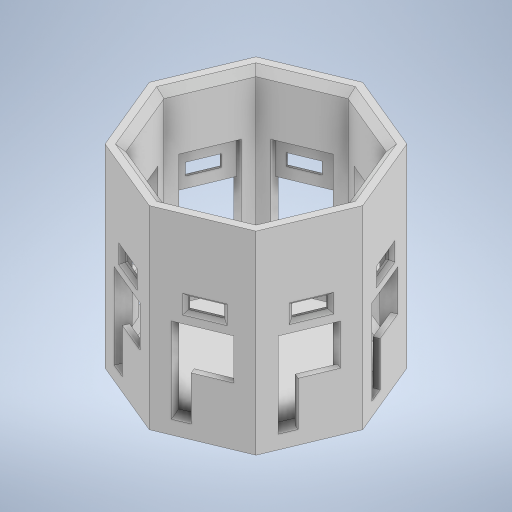
# Autodesk Inventor part: body_main
Saved by Autodesk Inventor 2023 (Build 270158000, 158)
## iProperties
Created: 2022-05-03
Part Number: body_main
Material: Ogólny
Document SubType Name: Modeling
Designer: Ciućmok
Density: 1 g/cm^3
Appearance: Domyślna
Author: Ciućmok
Autodesk Inventor part; units mm, degrees
ref_plane "YZ Plane" through (0, 0, 0) normal (1, 0, 0) x (0, 1, 0)
ref_plane "XZ Plane" through (0, 0, 0) normal (0, 1, 0) x (-1, 0, 0)
ref_plane "XY Plane" through (0, 0, 0) normal (0, 0, 1) x (1, 0, 0)
sketch "Szkic1" plane through (0, 0, 0) normal (0, 1, 0) x (-1, 0, 0)
  line L0 (0, 0) -> (0, 31.3575)
  line L1 (0, 31.3575) -> (22.1731, 22.1731)
  line L2 (22.1731, 22.1731) -> (0, 0)
  dimension "d0" = 45
  dimension "d1" = 24
  constraints: 6 end point, 1 equal length, 1 vertical
  measures "d0" angle of L2 L0
  measures "d1" distance of L0.end L1.end
extrude "Wyciągnięcie proste1" add sketch "Szkic1" along normal blind 2
sketch "Szkic2" plane through (0, 2, 0) normal (0, 1, 0) x (1, 0, 0)
  line L0 (-22.1731, -22.1731) -> (0, -31.3575) projected
  line L1 (0, 0) -> (-22.1731, -22.1731) projected
  line L2 (-19.1116, -19.1116) -> (0, -27.0279)
  line L3 (0, -31.3575) -> (0, 0) projected
  line L4 (0, -27.0279) -> (0, -31.3575)
  line L5 (-22.1731, -22.1731) -> (0, -31.3575)
  line L6 (-22.1731, -22.1731) -> (-19.1116, -19.1116)
  dimension "d4" = 4
  constraints: 8 end point, 2 point on line, 1 collinear, 1 parallel
  measures "d4" distance between parallel lines of L0 L2
extrude "Wyciągnięcie proste2" add sketch "Szkic2" along normal blind 40 contours L1 L2 L3 L0
sketch "Szkic3" plane through (-19.1116, 2, 19.1116) normal (0.3826834, 0, -0.9238795) x (-0.9238795, 0, -0.3826834)
  line L0 (-3.3304, 38) -> (-17.3304, 38)
  line L1 (-17.3304, 38) -> (-17.3304, 2)
  line L2 (-17.3304, 2) -> (-3.3304, 2)
  line L3 (-3.3304, 2) -> (-3.3304, 38)
  line L4 (1.6569, 40) -> (-22.3431, 40) construction
  line L5 (-20.6863, 0) -> (-10.3431, 0) construction
  line L6 (0.0255, 40) -> (-20.6863, 0) construction
  line L7 (-10.3431, 0) -> (0, 0) construction
  line L8 (0, 0) -> (-20.6863, 40) construction
  line L9 (-17.3304, 2) -> (-3.3304, 38) construction
  line L10 (-3.3304, 2) -> (-17.3304, 38) construction
  point P0 (-10.3431, -2)
  point P1 (-10.3304, 20)
  dimension "d7" = 14
  dimension "d8" = 36
  constraints: 16 end point, 2 midpoint, 2 parallel, 2 point on line, 1 horizontal, 1 perpendicular
  measures "d7" distance of L1.end L2.end
  measures "d8" distance of L0.end L1.end
sketch "Szkic4" plane through (0, 42, 0) normal (0, 1, 0) x (1, 0, 0)
  point P0 (0, 0)
sketch "Szkic5" plane through (0, 42, 0) normal (0, 1, 0) x (1, 0, 0)
  line L0 (0, -27.0279) -> (-19.1116, -19.1116) construction
  line L1 (-19.1116, -19.1116) -> (-22.1731, -22.1731) construction
  line L2 (-22.1731, -22.1731) -> (0, -31.3575) construction
  line L3 (0, -31.3575) -> (0, -27.0279) construction
  line L4 (-8.0251, -23.7038) -> (-9.5558, -27.3994) construction
  line L5 (-22.1731, -22.1731) -> (0, -31.3575) construction
  point P0 (0, 0)
  constraints: 2 end point, 2 point on line, 1 perpendicular
extrude "Wyciągnięcie proste3" cut sketch "Szkic3" against normal blind 2.4
sketch "Szkic6" plane through (-20.0301, 2, 21.329) normal (0.3826834, 0, -0.9238795) x (-0.9238795, 0, -0.3826834)
  line L0 (-17.3304, 2) -> (-17.3304, 38) projected
  line L1 (-3.3304, 2) -> (-17.3304, 2) projected
  line L2 (-3.3304, 38) -> (-3.3304, 2) projected
  line L3 (-17.3304, 38) -> (-3.3304, 38) projected
  line L4 (-3.3304, 38) -> (-3.3304, 2) projected
  line L5 (-17.3304, 38) -> (-3.3304, 38) projected
  line L6 (-7.7929, 2) -> (-7.7929, 27)
  line L7 (-7.7929, 27) -> (-3.3304, 27)
  line L8 (-7.7929, 27) -> (-17.3304, 27)
  line L9 (-17.3304, 2) -> (-17.3304, 38) projected
  line L10 (-17.3304, 15) -> (-7.7929, 15)
  point P0 (-10.3431, -2)
  point P1 (-17.3304, 25)
  point P2 (-17.3304, 13)
  point P3 (-3.3304, 27)
  dimension "d17" = 25
  dimension "d18" = 13
  constraints: 8 end point, 8 point on line, 2 perpendicular, 1 vertical
  measures "d17" distance of L6.start L6.end
  measures "d18" distance between parallel lines of L1 L10
extrude "Wyciągnięcie proste4" cut sketch "Szkic6" against normal through all contours L0 L8 L6 L10 | L6 L7 L2 L1
sketch "Szkic7" plane through (-20.0301, 2, 21.329) normal (0.3826834, 0, -0.9238795) x (-0.9238795, 0, -0.3826834)
  line L0 (-14.8304, 30.2) -> (-6.8304, 30.2)
  line L1 (-6.8304, 30.2) -> (-6.8304, 33.7)
  line L2 (-6.8304, 33.7) -> (-14.8304, 33.7)
  line L3 (-14.8304, 33.7) -> (-14.8304, 30.2)
  line L4 (-17.3304, 38) -> (-3.3304, 38) projected
  line L5 (-17.3304, 2) -> (-17.3304, 38) projected
  point P0 (-10.3431, -2)
  point P1 (-10.3304, 38)
  dimension "d19" = 8
  dimension "d20" = 3.5
  dimension "d21" = 4.3
  dimension "d22" = 2.5
  constraints: 8 end point, 2 parallel, 1 horizontal, 1 midpoint, 1 perpendicular
  measures "d19" distance of L2.end L1.end
  measures "d20" distance of L0.end L1.end
  measures "d21" distance from line of point (-10.33, 38) L2
  measures "d22" distance between parallel lines of L5 L3
extrude "Wyciągnięcie proste5" cut sketch "Szkic7" against normal blind 10
chamfer "Faza1" distance 1 angle 45 4 edges at (-10.6364, 35.7, 26.9518) (-14.3319, 33.95, 25.421) (-10.6364, 32.2, 26.9518) (-6.9409, 33.95, 28.4825)
pattern_circular "Szyk kołowy1" count 8 over 360 about axis through (0, 0, 0) along (0, 1, 0)
sketch "Szkic8" plane through (0, 42, 0) normal (0, 1, 0) x (1, 0, 0)
  line L0 (-22.1731, -22.1731) -> (0, -31.3575) projected
  line L1 (0, -31.3575) -> (22.1731, -22.1731) projected
  line L2 (22.1731, -22.1731) -> (31.3575, 0) projected
  line L3 (31.3575, 0) -> (22.1731, 22.1731) projected
  line L4 (22.1731, 22.1731) -> (0, 31.3575) projected
  line L5 (0, 31.3575) -> (-22.1731, 22.1731) projected
  line L6 (-22.1731, 22.1731) -> (-31.3575, 0) projected
  line L7 (-31.3575, 0) -> (-22.1731, -22.1731) projected
  line L8 (-19.1116, -19.1116) -> (-27.0279, 0) projected
  line L9 (-27.0279, 0) -> (-19.1116, 19.1116) projected
  line L10 (-19.1116, 19.1116) -> (0, 27.0279) projected
  line L11 (0, 27.0279) -> (19.1116, 19.1116) projected
  line L12 (19.1116, 19.1116) -> (27.0279, 0) projected
  line L13 (27.0279, 0) -> (19.1116, -19.1116) projected
  line L14 (19.1116, -19.1116) -> (0, -27.0279) projected
  line L15 (0, -27.0279) -> (-19.1116, -19.1116) projected
  point P0 (0, 0)
extrude "Wyciągnięcie proste6" add sketch "Szkic8" along normal blind 15
chamfer "Faza2" distance 2 angle 45 8 edges at (-9.5558, 57, 23.0698) (-23.0698, 57, 9.5558) (-23.0698, 57, -9.5558) (-9.5558, 57, -23.0698) (9.5558, 57, -23.0698) (23.0698, 57, -9.5558) (23.0698, 57, 9.5558) (9.5558, 57, 23.0698)
